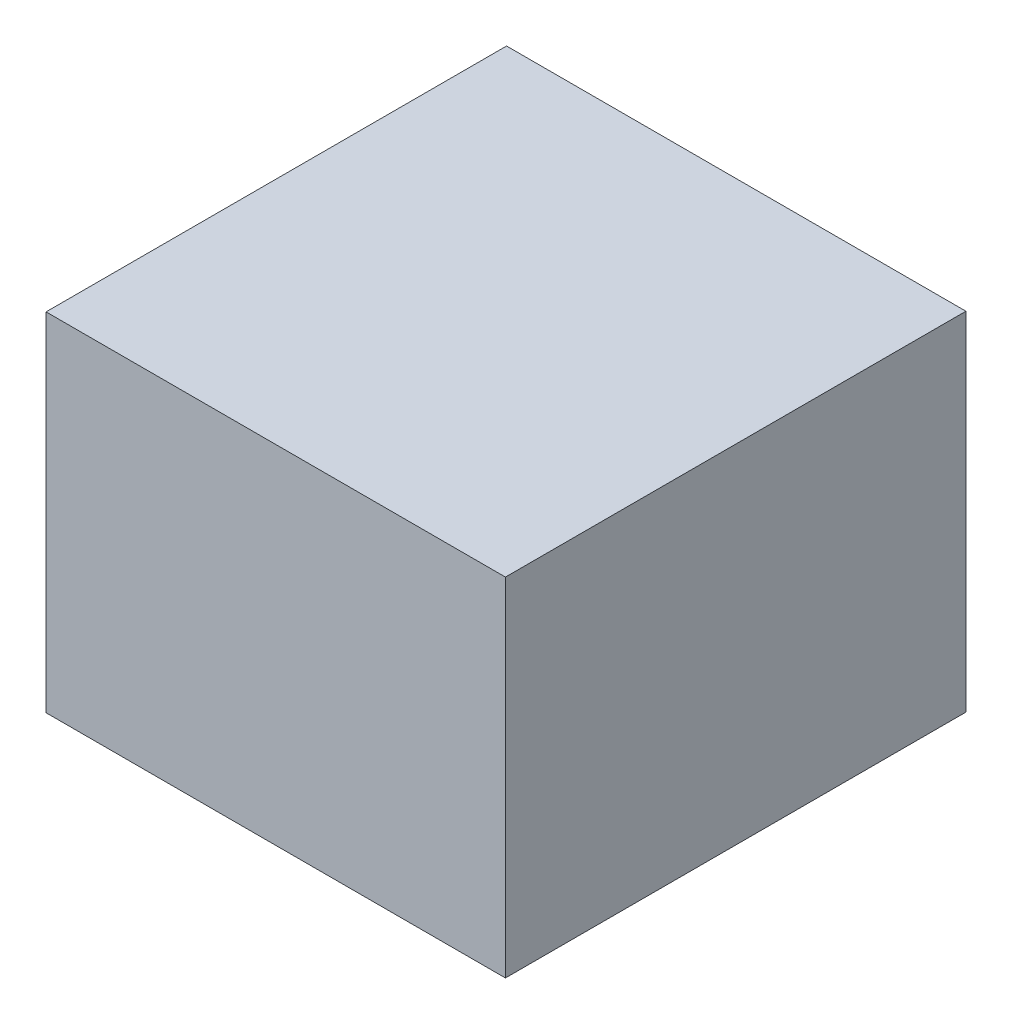
# Autodesk Inventor part: деталь будет крепить ремень
Saved by Autodesk Inventor 2024.2 (Build 282272000, 272)
## iProperties
Created: 2026-02-03
Part Number: деталь будет крепить ремень
Material: Типовые
Document SubType Name: Modeling
Designer: katya_notebook
Density: 1 g/cm^3
Appearance: По умолчанию
Author: katya_notebook
Autodesk Inventor part; units mm, degrees
ref_plane "YZ Plane" through (0, 0, 0) normal (1, 0, 0) x (0, 1, 0)
ref_plane "XZ Plane" through (0, 0, 0) normal (0, 1, 0) x (-1, 0, 0)
ref_plane "XY Plane" through (0, 0, 0) normal (0, 0, 1) x (1, 0, 0)
sketch "Эскиз1" plane through (0, 0, 0) normal (0, 0, 1) x (1, 0, 0)
  arc A0 (-2.4573, 6.775) -> (-3.0052, 7.2976) centre (-3.0114, 6.7426) ccw projected
  line L0 (-3.0052, 7.2976) -> (-3.0104, 6.025) projected
  line L1 (-3.0104, 6.025) -> (-3.0104, 5.7776) projected
  line L2 (-3.0104, 5.7776) -> (-1.0104, 5.7776) projected
  line L3 (-1.0104, 5.7776) -> (-1.0104, 6.1876) projected
  arc A1 (-1.0114, 6.1876) -> (-1.0104, 6.1876) centre (-1.0114, 6.7426) ccw projected
  line L4 (-1.0114, 6.1876) -> (-1.0114, 7.2976) projected
  arc A2 (-1.0114, 7.2976) -> (-1.5664, 6.7441) centre (-1.0114, 6.7426) ccw projected
  line L5 (-1.5664, 6.7441) -> (-1.5664, 6.7417) projected
  arc A3 (-1.5664, 6.7417) -> (-1.5647, 6.6993) centre (-1.0114, 6.7426) ccw projected
  arc A4 (-1.7142, 6.5376) -> (-1.5647, 6.6993) centre (-1.7142, 6.6876) ccw projected
  line L6 (-1.7142, 6.5376) -> (-2.3054, 6.5376) projected
  arc A5 (-2.4554, 6.6876) -> (-2.3054, 6.5376) centre (-2.3054, 6.6876) ccw projected
  line L7 (-2.4554, 6.6876) -> (-2.4554, 6.775) projected
  line L8 (-2.4554, 6.775) -> (-2.4573, 6.775) projected
  arc A6 (-0.4635, 6.775) -> (-1.0114, 7.2976) centre (-1.0175, 6.7426) ccw projected
  line L9 (-1.0114, 7.2976) -> (-1.0166, 6.025) projected
  line L10 (-1.0166, 6.025) -> (-1.0166, 5.7776) projected
  line L11 (-1.0166, 5.7776) -> (0.9834, 5.7776) projected
  line L12 (0.9834, 5.7776) -> (0.9834, 6.1876) projected
  arc A7 (0.9825, 6.1876) -> (0.9834, 6.1876) centre (0.9825, 6.7426) ccw projected
  line L13 (0.9825, 6.1876) -> (0.9825, 7.2976) projected
  arc A8 (0.9825, 7.2976) -> (0.4275, 6.7441) centre (0.9825, 6.7426) ccw projected
  line L14 (0.4275, 6.7441) -> (0.4275, 6.7417) projected
  arc A9 (0.4275, 6.7417) -> (0.4291, 6.6993) centre (0.9825, 6.7426) ccw projected
  arc A10 (0.2796, 6.5376) -> (0.4291, 6.6993) centre (0.2796, 6.6876) ccw projected
  line L15 (0.2796, 6.5376) -> (-0.3116, 6.5376) projected
  arc A11 (-0.4616, 6.6876) -> (-0.3116, 6.5376) centre (-0.3116, 6.6876) ccw projected
  line L16 (-0.4616, 6.6876) -> (-0.4616, 6.775) projected
  line L17 (-0.4616, 6.775) -> (-0.4635, 6.775) projected
  arc A12 (1.5304, 6.775) -> (0.9825, 7.2976) centre (0.9763, 6.7426) ccw projected
  line L18 (0.9825, 7.2976) -> (0.9772, 6.025) projected
  line L19 (0.9772, 6.025) -> (0.9772, 5.7776) projected
  line L20 (0.9772, 5.7776) -> (2.9772, 5.7776) projected
  line L21 (2.9772, 5.7776) -> (2.9772, 6.1876) projected
  arc A13 (2.9763, 6.1876) -> (2.9772, 6.1876) centre (2.9763, 6.7426) ccw projected
  line L22 (2.9763, 6.1876) -> (2.9763, 7.2976) projected
  arc A14 (2.9763, 7.2976) -> (2.4213, 6.7441) centre (2.9763, 6.7426) ccw projected
  line L23 (2.4213, 6.7441) -> (2.4213, 6.7417) projected
  arc A15 (2.4213, 6.7417) -> (2.423, 6.6993) centre (2.9763, 6.7426) ccw projected
  arc A16 (2.2734, 6.5376) -> (2.423, 6.6993) centre (2.2734, 6.6876) ccw projected
  line L24 (2.2734, 6.5376) -> (1.6822, 6.5376) projected
  arc A17 (1.5322, 6.6876) -> (1.6822, 6.5376) centre (1.6822, 6.6876) ccw projected
  line L25 (1.5322, 6.6876) -> (1.5322, 6.775) projected
  line L26 (1.5322, 6.775) -> (1.5304, 6.775) projected
  arc A18 (3.5242, 6.775) -> (2.9763, 7.2976) centre (2.9701, 6.7426) ccw projected
  line L27 (2.9763, 7.2976) -> (2.9711, 6.025) projected
  line L28 (2.9711, 6.025) -> (2.9711, 5.7776) projected
  line L29 (2.9711, 5.7776) -> (4.9711, 5.7776) projected
  line L30 (4.9711, 5.7776) -> (4.9711, 6.1876) projected
  arc A19 (4.9701, 6.1876) -> (4.9711, 6.1876) centre (4.9701, 6.7426) ccw projected
  line L31 (4.9701, 6.1876) -> (4.9701, 7.2976) projected
  arc A20 (4.9701, 7.2976) -> (4.4151, 6.7441) centre (4.9701, 6.7426) ccw projected
  line L32 (4.4151, 6.7441) -> (4.4151, 6.7417) projected
  arc A21 (4.4151, 6.7417) -> (4.4168, 6.6993) centre (4.9701, 6.7426) ccw projected
  arc A22 (4.2673, 6.5376) -> (4.4168, 6.6993) centre (4.2673, 6.6876) ccw projected
  line L33 (4.2673, 6.5376) -> (3.6761, 6.5376) projected
  arc A23 (3.5261, 6.6876) -> (3.6761, 6.5376) centre (3.6761, 6.6876) ccw projected
  line L34 (3.5261, 6.6876) -> (3.5261, 6.775) projected
  line L35 (3.5261, 6.775) -> (3.5242, 6.775) projected
  line L36 (4.9701, 7.2976) -> (4.9701, 8.7976)
  line L37 (4.9701, 8.7976) -> (-3.0052, 8.7976)
  line L38 (-3.0052, 7.2976) -> (4.9701, 7.2976)
  line L39 (-3.0052, 8.7976) -> (-3.0052, 7.2976)
  line L40 (-3.0052, 5.7776) -> (4.9701, 5.7776)
  line L41 (4.9701, 5.7776) -> (4.9701, 4.2776)
  line L42 (4.9701, 4.2776) -> (-3.0052, 4.2776)
  line L43 (-3.0052, 4.2776) -> (-3.0052, 5.7776)
  line L44 (4.9701, 5.0276) -> (-5.8657, 5.0276)
  arc A24 (-3.0052, 2.7576) -> (-2.4573, 3.2802) centre (-3.0114, 3.3126) ccw
  line L45 (-3.0052, 2.7576) -> (-3.0104, 4.0302)
  line L46 (-3.0104, 4.0302) -> (-3.0104, 4.2776)
  line L47 (-1.0104, 4.2776) -> (-1.0104, 3.8676)
  arc A25 (-1.0104, 3.8676) -> (-1.0114, 3.8676) centre (-1.0114, 3.3126) ccw
  line L48 (-1.0114, 3.8676) -> (-1.0114, 2.7576)
  arc A26 (-1.5664, 3.311) -> (-1.0114, 2.7576) centre (-1.0114, 3.3126) ccw
  line L49 (-1.5664, 3.311) -> (-1.5664, 3.3135)
  arc A27 (-1.5647, 3.3559) -> (-1.5664, 3.3135) centre (-1.0114, 3.3126) ccw
  arc A28 (-1.5647, 3.3559) -> (-1.7142, 3.5176) centre (-1.7142, 3.3676) ccw
  line L50 (-1.7142, 3.5176) -> (-2.3054, 3.5176)
  arc A29 (-2.3054, 3.5176) -> (-2.4554, 3.3676) centre (-2.3054, 3.3676) ccw
  line L51 (-2.4554, 3.3676) -> (-2.4554, 3.2802)
  line L52 (-2.4554, 3.2802) -> (-2.4573, 3.2802)
  arc A30 (-1.0114, 2.7576) -> (-0.4635, 3.2802) centre (-1.0175, 3.3126) ccw
  line L53 (-1.0114, 2.7576) -> (-1.0166, 4.0302)
  line L54 (-1.0166, 4.0302) -> (-1.0166, 4.2776)
  line L55 (0.9834, 4.2776) -> (0.9834, 3.8676)
  arc A31 (0.9834, 3.8676) -> (0.9825, 3.8676) centre (0.9825, 3.3126) ccw
  line L56 (0.9825, 3.8676) -> (0.9825, 2.7576)
  arc A32 (0.4275, 3.311) -> (0.9825, 2.7576) centre (0.9825, 3.3126) ccw
  line L57 (0.4275, 3.311) -> (0.4275, 3.3135)
  arc A33 (0.4291, 3.3559) -> (0.4275, 3.3135) centre (0.9825, 3.3126) ccw
  arc A34 (0.4291, 3.3559) -> (0.2796, 3.5176) centre (0.2796, 3.3676) ccw
  line L58 (0.2796, 3.5176) -> (-0.3116, 3.5176)
  arc A35 (-0.3116, 3.5176) -> (-0.4616, 3.3676) centre (-0.3116, 3.3676) ccw
  line L59 (-0.4616, 3.3676) -> (-0.4616, 3.2802)
  line L60 (-0.4616, 3.2802) -> (-0.4635, 3.2802)
  arc A36 (0.9825, 2.7576) -> (1.5304, 3.2802) centre (0.9763, 3.3126) ccw
  line L61 (0.9825, 2.7576) -> (0.9772, 4.0302)
  line L62 (0.9772, 4.0302) -> (0.9772, 4.2776)
  line L63 (2.9772, 4.2776) -> (2.9772, 3.8676)
  arc A37 (2.9772, 3.8676) -> (2.9763, 3.8676) centre (2.9763, 3.3126) ccw
  line L64 (2.9763, 3.8676) -> (2.9763, 2.7576)
  arc A38 (2.4213, 3.311) -> (2.9763, 2.7576) centre (2.9763, 3.3126) ccw
  line L65 (2.4213, 3.311) -> (2.4213, 3.3135)
  arc A39 (2.423, 3.3559) -> (2.4213, 3.3135) centre (2.9763, 3.3126) ccw
  arc A40 (2.423, 3.3559) -> (2.2734, 3.5176) centre (2.2734, 3.3676) ccw
  line L66 (2.2734, 3.5176) -> (1.6822, 3.5176)
  arc A41 (1.6822, 3.5176) -> (1.5322, 3.3676) centre (1.6822, 3.3676) ccw
  line L67 (1.5322, 3.3676) -> (1.5322, 3.2802)
  line L68 (1.5322, 3.2802) -> (1.5304, 3.2802)
  arc A42 (2.9763, 2.7576) -> (3.5242, 3.2802) centre (2.9701, 3.3126) ccw
  line L69 (2.9763, 2.7576) -> (2.9711, 4.0302)
  line L70 (2.9711, 4.0302) -> (2.9711, 4.2776)
  line L71 (4.9711, 4.2776) -> (4.9711, 3.8676)
  arc A43 (4.9711, 3.8676) -> (4.9701, 3.8676) centre (4.9701, 3.3126) ccw
  line L72 (4.9701, 3.8676) -> (4.9701, 2.7576)
  arc A44 (4.4151, 3.311) -> (4.9701, 2.7576) centre (4.9701, 3.3126) ccw
  line L73 (4.4151, 3.311) -> (4.4151, 3.3135)
  arc A45 (4.4168, 3.3559) -> (4.4151, 3.3135) centre (4.9701, 3.3126) ccw
  arc A46 (4.4168, 3.3559) -> (4.2673, 3.5176) centre (4.2673, 3.3676) ccw
  line L74 (4.2673, 3.5176) -> (3.6761, 3.5176)
  arc A47 (3.6761, 3.5176) -> (3.5261, 3.3676) centre (3.6761, 3.3676) ccw
  line L75 (3.5261, 3.3676) -> (3.5261, 3.2802)
  line L76 (3.5261, 3.2802) -> (3.5242, 3.2802)
  line L77 (4.9701, 2.7576) -> (-3.0052, 2.7576)
  line L78 (-3.0052, 2.7576) -> (-3.0052, 1.2576)
  line L79 (-3.0052, 1.2576) -> (4.9701, 1.2576)
  line L80 (4.9701, 1.2576) -> (4.9701, 2.7576)
  point P0 (0, 0)
  point P1 (-3.0052, 8.0476)
  point P2 (-3.0052, 5.0276)
  point P3 (4.9701, 8.0476)
  point P4 (4.9701, 5.7776)
  point P5 (-3.5365, 6.9641)
  point P6 (-1.5427, 6.9641)
  point P7 (0.4512, 6.9641)
  point P8 (2.445, 6.9641)
  point P9 (0.4512, 3.5359)
  point P10 (-1.5427, 3.5359)
  point P11 (-3.5365, 3.5359)
  point P12 (-3.0052, 2.7576)
  point P13 (2.445, 3.5359)
  dimension "d0" = 1.5
  dimension "d1" = 0
  constraints: 90 end point, 85 symmetric about line, 48 point on circle, 24 centre point, 4 equal length, 4 horizontal, 4 midpoint, 4 parallel, 3 perpendicular, 2 vertical, 2 vertical alignment, 24 other
  measures "d0" distance between parallel lines of L37 L38
  measures "d1" distance between parallel lines of L2 L40
extrude "Выдавливание1" add sketch "Эскиз1" along normal blind 8 contours A0 L38 A1 A4 L6 A5 L7 | L39 L37 L36 L38 | L38 A7 A10 L15 A11 A1 | L38 A13 A16 L24 A17 A7 | L2 L11 L20 L29 L41 L44 L43 | L38 A19 A22 L33 A23 A13 | L44 L41 L42 L43 | A43 L77 A37 A47 L74 A46 | L80 L79 L78 L77 | A35 L58 A34 A31 L77 A25 | L77 A24 L51 A29 L50 A28 A25 | L77 A31 A41 L66 A40 A37
sketch "Эскиз2" plane through (4.9701, 4.2776, 0) normal (1, 0, 0) x (0, 0, -1)
  line L0 (0, -1.52) -> (0, -3.02) projected
  line L1 (-8, 3.02) -> (-8, 4.52) projected
  line L2 (0, -3.02) -> (-8, -3.02)
  line L3 (-8, -3.02) -> (-8, 4.52)
  line L4 (-8, 4.52) -> (0, 4.52)
  line L5 (0, 4.52) -> (0, -3.02)
  point P0 (0, -4.2776)
  point P1 (0, -1.52)
  point P2 (-8, 3.02)
  constraints: 8 end point, 2 parallel, 1 horizontal, 1 perpendicular
extrude "Выдавливание2" add sketch "Эскиз2" along normal blind 2
sketch "Эскиз3" plane through (0, 0, 8) normal (0, 0, 1) x (1, 0, 0)
  line L0 (-3.0052, 1.2576) -> (6.9701, 1.2576) projected
  line L1 (-3.0052, 8.7976) -> (6.9701, 8.7976) projected
  line L2 (6.9701, 1.2576) -> (-3.0052, 1.2576)
  line L3 (-3.0052, 1.2576) -> (-3.0052, 8.7976)
  line L4 (-3.0052, 8.7976) -> (6.9701, 8.7976)
  line L5 (6.9701, 8.7976) -> (6.9701, 1.2576)
  point P0 (0, 0)
  point P1 (-3.0052, 1.2576)
  point P2 (6.9701, 8.7976)
  constraints: 8 end point, 2 parallel, 1 horizontal, 1 perpendicular
extrude "Выдавливание3" add sketch "Эскиз3" along normal blind 2
